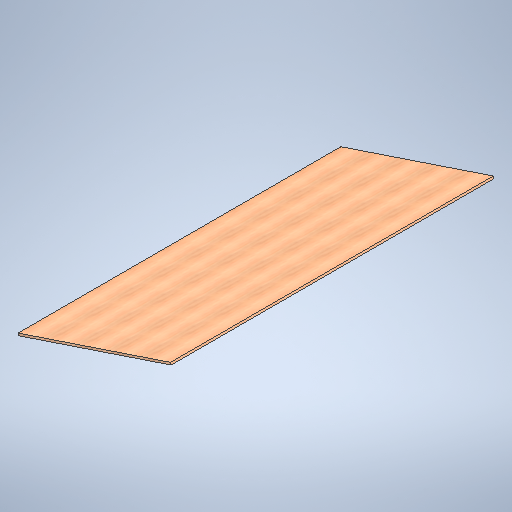
# Autodesk Inventor part: OSB_For_Rear_Roof
Saved by Autodesk Inventor 2025.1 (Build 291241020, 241B)
## iProperties
Created: 2024-09-15
Part Number: OSB_For_Rear_Roof
Material: Wood (Birch)
Document SubType Name: Modeling
Designer: Tom
Density: 0.55 g/cm^3
Appearance: Birch - Natural Polished
Author: Tom
Autodesk Inventor part; units mm, degrees
ref_plane "YZ Plane" through (0, 0, 0) normal (1, 0, 0) x (0, 1, 0)
ref_plane "XZ Plane" through (0, 0, 0) normal (0, 1, 0) x (-1, 0, 0)
ref_plane "XY Plane" through (0, 0, 0) normal (0, 0, 1) x (1, 0, 0)
sketch "Sketch1" plane through (0, 0, 0) normal (0, 0, 1) x (1, 0, 0)
  line L0 (0, 0) -> (3294.2276, 1099.144)
  line L1 (3294.2276, 1246.4151) -> (-135.0962, 102.1952)
  line L2 (0, 0) -> (-135.0962, 0)
  line L3 (-135.0962, 0) -> (-135.0962, 102.1952)
  line L4 (-135.0962, 102.1952) -> (1593.1098, 678.8242)
  line L5 (3294.2276, 1099.144) -> (3263.9, 1099.144)
  line L6 (3294.2276, 1099.144) -> (3294.2276, 1246.4151)
  line L7 (-88.9, 0) -> (-88.9, 117.6089)
  line L8 (3263.9, 1089.025) -> (3263.9, 1236.2961)
  line L9 (-135.0962, 102.1952) -> (-135.0962, 118.9305)
  line L10 (-135.0962, 118.9305) -> (1016.4014, 503.1364)
  line L11 (1016.4014, 503.1364) -> (1021.4259, 488.0776)
  line L12 (1021.4259, 488.0776) -> (-135.0962, 102.1952)
  dimension "d5" = 139.7
  dimension "d17" = 88.9
  dimension "d19" = 3352.8
  dimension "d23" = 30.3276
  dimension "d28" = 46.1962
  dimension "d33" = 1089.025
  dimension "d36" = 15.875
  dimension "d37" = 1219.2
  constraints: 26 end point, 6 point on line, 5 vertical, 2 coincident, 2 horizontal, 2 parallel, 1 collinear, 1 perpendicular
  measures "d5" distance between parallel lines of L1 L0
  measures "d17" distance from line of L7 point (0, 0)
  measures "d19" distance between parallel lines of L7 L8
  measures "d23" distance between parallel lines of L6 L8
  measures "d28" distance between parallel lines of L3 L7
  measures "d33" vertical distance of L8.start point (0, 0)
  measures "d36" distance between parallel lines of L10 L1
  measures "d37" distance of L11.end L1.end
extrude "Extrusion2" add sketch "Sketch1" along normal blind 2438.4 contours L1 L9 L10 L11
body "Solid2"
